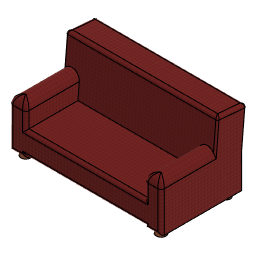
sohva v3 (Autodesk Fusion 360 design; units mm, degrees)
Autodesk Fusion 360 part; units mm, degrees
note: some values were not read from the file. Chosen so that the rebuilt part matches the saved one: which bodies a step acts on. Set by a fixed rule: which face or edge a step refers to.
sketch "Sketch1" plane through (0, 0, 0) normal (0, 0, 1) x (1, 0, 0) in component "penkki"
  line L0 (-20, 10) -> (20, 10)
  line L1 (20, 10) -> (20, -15)
  line L2 (20, -15) -> (-20, -15)
  line L3 (-20, -15) -> (-20, 10)
  constraint horizontal L0
  constraint vertical L1
  constraint horizontal L2
  constraint vertical L3
extrude "Extrude1" add sketch "Sketch1" along normal blind 5 makes body 1 in component "penkki"
sketch "Sketch1 (2)" plane through (0, 0, 0) normal (0, 0, 1) x (1, 0, 0) in component "jalkatuki"
  circle A0 centre (-29.6421, 8.6291) radius 1.5
  dimension "d8" = 3
  measures "d8" diameter of A0
extrude "Extrude1'" add sketch "Sketch1 (2)" along normal blind 3 separate body makes body 2 in component "jalkatuki"
copy_body "CopyPasteBodies1" bodies 2 makes body 3 in component "jalkatuki"
move_body "Move1" bodies 3 to x (1, 0, 0) y (0, 1, 0) z (0, 0, 1) at (-15, 0, 0) in component "jalkatuki"
sketch "Sketch2" plane through (0, 0, 5) normal (0, 0, 1) x (-1, 0, 0) in component "jalkatuki"
  line L0 (20, 15) -> (-20, 15)
  line L1 (-20, 15) -> (-20, -10)
  line L2 (-20, -10) -> (20, -10)
  line L3 (20, -10) -> (20, 15)
  line L4 (65, -5) -> (40, -5)
  line L5 (40, -5) -> (40, 0)
  line L6 (40, 0) -> (65, 0)
  line L7 (65, 0) -> (65, -5)
  constraint horizontal L4
  constraint vertical L5
  constraint horizontal L6
  constraint vertical L7
extrude "Extrude2" add sketch "Sketch2" along normal blind 15 separate body contours L4 L5 L6 L7 makes body 4 in component "jalkatuki"
fillet "Fillet1" radius 2.5 1 faces at (-56.6667, 3.3333, 20) on bodies 4 in component "jalkatuki"
move_body "Move2" bodies 2 to x (1, 0, 0) y (0, 1, 0) z (0, 0, 1) at (-3.9761, -0.7905, 0) in component "jalkatuki"
move_body "Move3" bodies 3 to x (1, 0, 0) y (0, 1, 0) z (0, 0, 1) at (0.1193, -0.527, 0) in component "jalkatuki"
move_body "Move4" bodies 3 to x (1, 0, 0) y (0, 1, 0) z (0, 0, 1) at (-9.8807, 0.1317, 0) in component "jalkatuki"
combine "Combine1" operation add target body 4 tool bodies 2 makes body 5 at (-33.1405, 9.2606, 1) in component "jalkatuki"
move_body "Move5" bodies 3 to x (1, 0, 0) y (0, 1, 0) z (0, 0, 1) at (0, 5.461, 3.3892) in component "jalkatuki"
move_body "Move6" bodies 3 to x (1, 0, 0) y (0, 1, 0) z (0, 0, 1) at (-7, -16, 0) in component "jalkatuki"
move_body "Move7" bodies 5 to x (1, 0, 0) y (0, 1, 0) z (0, 0, 1) at (-9, -9.9, 0) in component "jalkatuki"
move_body "Move8" bodies 3 to x (1, 0, 0) y (0, 1, 0) z (0, 0, 1) at (0, 0.1, 0) in component "jalkatuki"
move_body "Move9" bodies 3 to x (1, 0, 0) y (0, 1, 0) z (0, 0, 1) at (0, -0.35, 0) in component "jalkatuki"
move_body "Move10" bodies 5 to x (1, 0, 0) y (0, 1, 0) z (0, 0, 1) at (0, -0.45, 0) in component "jalkatuki"
move_body "Move11" bodies 3 to x (1, 0, 0) y (0, 1, 0) z (0, 0, 1) at (-0.9, 0, 0) in component "jalkatuki"
move_body "Move12" bodies 3 to x (1, 0, 0) y (0, 1, 0) z (0, 0, 1) at (0, 0.1, 0) in component "jalkatuki"
move_body "Move13" bodies 3 to x (1, 0, 0) y (0, 1, 0) z (0, 0, 1) at (0, -0.05, 0) in component "jalkatuki"
move_body "Move14" bodies 4 to x (1, 0, 0) y (0, 1, 0) z (0, 0, 1) at (0, -4.7, 0) in component "jalkatuki"
move_body "Move15" bodies 4 to x (1, 0, 0) y (0, 1, 0) z (0, 0, 1) at (0, -0.2, 0) in component "jalkatuki"
move_body "Move16" bodies 4 to x (1, 0, 0) y (0, 1, 0) z (0, 0, 1) at (0, -0.1, 0) in component "jalkatuki"
move_body "Move17" bodies 5 to x (1, 0, 0) y (0, 1, 0) z (0, 0, 1) at (0, 0, 3.4) in component "jalkatuki"
move_body "Align1" bodies 3 to x (1, 0, 0) y (0, 1, 0) z (0, 0, 1) at (19.6853, -0.0062, 0.0108) in component "jalkatuki"
move_body "Move18" bodies 3 to x (1, 0, 0) y (0, 1, 0) z (0, 0, 1) at (-20, 0, 0) in component "jalkatuki"
move_body "Align2" bodies 4 to x (1, 0, 0) y (0, 1, 0) z (0, 0, 1) at (-10.1182, -0.0113, -8.8136) in component "jalkatuki"
move_body "Move19" bodies 4 to x (1, 0, 0) y (0, 1, 0) z (0, 0, 1) at (10, 0, 8.7) in component "jalkatuki"
combine "Combine2" operation add target body 5 tool bodies 4 in component "jalkatuki"
combine "Combine3" operation add target body 5 tool bodies 3 in component "jalkatuki"
move_face "OffsetFaces1" offset 2 1 faces at (-6.6667, 1.6667, 0) on bodies 1 in component "penkki"
copy_body "CopyPasteBodies1'" bodies 5 body 5 seen with x (0, -1, 0) y (1, 0, 0) z (0, 0, 1) at (-18.4887, -55.1182, -7.5082) makes body 6 in component "penkki"
copy_body "CopyPasteBodies2" bodies 5 body 5 seen with x (0, -1, 0) y (1, 0, 0) z (0, 0, 1) at (23.5113, -55.1182, -7.5082) makes body 7 in component "penkki"
combine "Combine1'" operation add target body 1 tool bodies 6 in component "penkki"
combine "Combine2'" operation add target body 1 tool bodies 7 in component "penkki"
sketch "Sketch1 (3)" plane through (0, 0, 0) normal (0, 0, 1) x (1, 0, 0) in component "Component"
  line L0 (0, 5) -> (47, 5)
  line L1 (47, 5) -> (47, 0)
  line L2 (47, 0) -> (0, 0)
  line L3 (0, 0) -> (0, 5)
  dimension "d15" = 47
  dimension "d16" = 5
  constraint horizontal L0
  constraint vertical L1
  constraint horizontal L2
  constraint vertical L3
  measures "d15" distance of L0.start L0.end
  measures "d16" distance of L0.start L2.end
extrude "Extrude1''" add sketch "Sketch1 (3)" along normal blind 20 separate body makes body 8 in component "Component"
move_body "Move1'" bodies 8 to x (1, 0, 0) y (0, 1, 0) z (0, 0, 1) at (0, 12, 0) in component "Component"
move_body "Move2'" bodies 8 to x (1, 0, 0) y (0, 0.984808, 0.173648) z (0, -0.173648, 0.984808) at (0, 2.1519, -9.7365) in component "Component"
move_body "Move3'" bodies 8 to x (1, 0, 0) y (0, 0.996195, -0.087156) z (0, 0.087156, 0.996195) at (0, -1.2931, 0.8857) in component "Component"
move_body "Move4'" bodies 8 to x (1, 0, 0) y (0, 1, 0) z (0, 0, 1) at (0, -0.2, 0) in component "Component"
move_face "OffsetFaces1'" offset 4 1 faces at (15.6667, 10.5943, 5.3272) on bodies 8 in component "Component"
fillet "Fillet1'" radius 1 1 faces at (15.6667, 13.7488, -7.7811) on bodies 8 in component "Component"
fillet "Fillet2" radius 0.5 9 faces at (47, 13.1096, -0.4757) (46.1073, 11.0723, -8.0094) (16, 13.4167, -7.8101) (31, 8.6407, -8.2199) (15.6667, 6.5805, 5.3106) (0.8927, 11.0723, -8.0094) (0, 13.1096, -0.4757) (15.9194, 16.0982, -7.5065) (31.3333, 16.0982, -0.2142) on bodies 8 in component "Component"
fillet "Fillet1''" radius 1 3 faces at (6.1667, 10, 2.6667) (-20.6229, 8.8336, 11.993) (21.3771, 8.8336, 11.993) on bodies 1 in component "penkki"
move_body "Move5'" bodies 8 to x (1, 0, 0) y (0, 1, 0) z (0, 0, 1) at (0, -0.2, 0) in component "Component"
combine "Combine3'" operation add target body 1 tool bodies 8 body 8 seen with x (1, 0, 0) y (0, -1, 0) z (0, 0, -1) at (-23.5, 0, 12.5802) in component "penkki"
move_body "Move1''" bodies 1 to x (1, 0, 0) y (0, 1, 0) z (0, 0, 1) at (0, 0, -1) in component "penkki"
component "penkki" placed x (-1, 0, 0) y (0, -1, 0) z (0, 0, 1) at (-33.6182, 12.9887, 7.5082)
component "Component" placed x (-1, 0, 0) y (0, 1, 0) z (0, 0, -1) at (-10.1182, 12.9887, 20.0884)
named bodies: "Body6"
